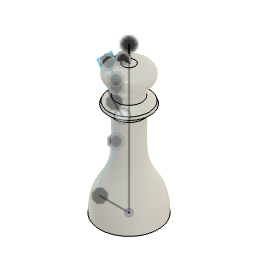
King v3 (Autodesk Fusion 360 design; units mm, degrees)
Autodesk Fusion 360 part; units mm, degrees
sketch "Sketch1" plane through (0, 0, 0) normal (0, 1, 0) x (1, 0, 0)
  line L0 (0, 0) -> (0, -100)
  line L1 (0, 0) -> (-20, 0)
  line L2 (-8.6434, -69.9212) -> (-13.6365, -66.5542)
  line L3 (-13.6365, -66.5542) -> (-14.3183, -64.9565)
  line L4 (-14.3183, -64.9565) -> (-4.481, -55.1193)
  spline S0 degree 5 poles (-4, -89) (-4.6763, -88.9623) (-5.9743, -88.8537) (-7.7573, -88.5916) (-9.8043, -88.0419) (-11.7956, -87.0232) (-13.199, -85.6887) (-13.9846, -84.0936) (-14.1422, -82.3218) (-13.6327, -80.5641) (-12.5746, -78.9465) (-11.248, -77.4692) (-9.9693, -76.0893) (-9.0179, -74.7445) (-8.5482, -73.3986) (-8.4819, -72.0855) (-8.5773, -71.1228) (-8.6309, -70.4847) (-8.6432, -70.102) (-8.6434, -69.9212) knots 0 0 0 0 0 0 0.066667 0.133333 0.2 0.266667 0.333333 0.4 0.466667 0.533333 0.6 0.666667 0.733333 0.8 0.866667 0.933333 1 1 1 1 1 1
  line L5 (-8.641, -71.8011) -> (-8.6458, -68.0414)
  line L6 (-14.1075, -84.4842) -> (-13.8758, -80.5449)
  line L7 (-4, -89) -> (0, -89)
  spline S1 degree 5 poles (-20, 0) (-20, -2.3229) (-19.8256, -6.6009) (-19.0404, -11.9147) (-17.1031, -17.0904) (-13.9997, -21.8824) (-11.1553, -26.7164) (-9.2779, -32.813) (-8.7086, -40.6017) (-8.6412, -48.2789) (-8.7525, -54.622) (-9.0569, -58.1731) (-9.4994, -59.8608) (-9.9098, -60.548) (-10.1437, -60.782) knots 0 0 0 0 0 0 0.1 0.2 0.3 0.4 0.5 0.6 0.7 0.8 0.9 1 1 1 1 1 1
  line L8 (-8.8945, -59.5327) -> (-11.393, -62.0312)
  line L9 (-20, 10.3262) -> (-20, -10.3262)
  line L10 (-9.6033, -30.4182) -> (-8.3967, -45.5818)
  line L11 (-12.3745, -78.8073) -> (-11.0265, -87.3321)
  line L12 (-12.3745, -78.8073) -> (-17.9409, -74.5687)
  line L13 (-11.0265, -87.3321) -> (-12.1499, -89.4521)
  line L14 (-12.1499, -89.4521) -> (-21.398, -80.2984)
  line L15 (-21.398, -80.2984) -> (-17.9409, -74.5687)
  point P0 (-13.9916, -82.5146)
  point P1 (-9.0226, -74.5163)
  point P2 (-9, -38)
  dimension "d1" = 100
  dimension "d2" = 20
  dimension "d3" = 45
  constraint coincident L0.start L1.start
  constraint vertical L0
  constraint perpendicular L0 L1
  constraint midpoint L2.start L5
  constraint midpoint P0 L6
  constraint coincident L0 L7.end
  constraint perpendicular L0 L7
  constraint coincident L4 S1.end
  constraint midpoint S1.end L8
  constraint parallel L4 L8
  constraint midpoint L1.end L9
  constraint perpendicular L1 L9
  constraint midpoint P2 L10
  constraint coincident S0 L11.end
  constraint coincident S0 L11.start
  measures "d1" distance of L0.start L0.end
  measures "d2" distance of L0.start L1.end
  measures "d3" angle of L0 L4
revolve "Revolve1" add sketch "Sketch1" angle 360 about axis through (0, 0, 0) along (0, 0, 1) contours L0 L1 L2 L3 L4 S0 L7 S1 L8 L11 | S0 L11
revolve "Revolve2" cut sketch "Sketch1" angle 30 about axis through (-12.3745, 0, 78.8073) along (-0.156176, 0, -0.987729) second angle 30 contours S0 L12 L13 L14 L15 | S0 L11
equation "d2 = 0.4 * d1 / 2"
